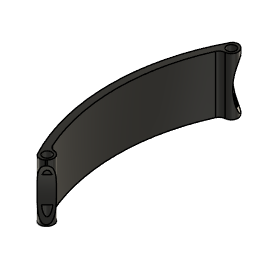
side_coverv6 (Autodesk Fusion 360 design; units mm, degrees)
Autodesk Fusion 360 part; units mm, degrees
note: some values were not read from the file. Set by a fixed rule: which sketch regions a step uses.
sketch "スケッチ1" plane through (0, 0, 2) normal (0, 0, 1) x (-1, 0, 0)
  arc A0 (6.6797, -60.2824) -> (7.9909, -61.0636) centre (8.2815, -59.0848) ccw
  arc A1 (37.5046, -75.2506) -> (7.9909, -61.0636) centre (0, -115.48) ccw
  arc A2 (37.555, -78.1277) -> (37.5046, -75.2506) centre (36.1408, -76.7135) ccw
  line L0 (37.555, -78.1277) -> (34.7247, -80.958)
  arc A3 (31.9509, -81.0106) -> (34.7247, -80.958) centre (33.3105, -79.5438) ccw
  arc A4 (31.9509, -81.0106) -> (-31.9509, -81.0106) centre (0, -115.48) ccw
  arc A5 (-34.7247, -80.958) -> (-31.9509, -81.0106) centre (-33.3105, -79.5438) ccw
  line L1 (-34.7247, -80.958) -> (-37.555, -78.1277)
  arc A6 (-37.5046, -75.2506) -> (-37.555, -78.1277) centre (-36.1408, -76.7135) ccw
  arc A7 (-7.9909, -61.0636) -> (-37.5046, -75.2506) centre (0, -115.48) ccw
  arc A8 (-7.9909, -61.0636) -> (-6.6797, -60.2824) centre (-8.2815, -59.0848) ccw
  arc A9 (-5.0779, -59.48) -> (-6.6797, -60.2824) centre (-5.0779, -61.48) ccw
  line L2 (-5.0779, -59.48) -> (5.0779, -59.48)
  arc A10 (6.6797, -60.2824) -> (5.0779, -59.48) centre (5.0779, -61.48) ccw
  arc A11 (80.8919, -35.1534) -> (72.8829, -37.1429) centre (78.5398, -42.7998) ccw
  line L3 (72.8829, -37.1429) -> (66.8393, -43.1865)
  arc A12 (62.5966, -43.1865) -> (66.8393, -43.1865) centre (64.7179, -41.0652) ccw
  line L4 (62.5966, -43.1865) -> (58.9846, -39.5745)
  arc A13 (58.6276, -32.9007) -> (58.9846, -39.5745) centre (62.5201, -36.039) ccw
  arc A14 (58.6276, -32.9007) -> (58.4491, -29.5638) centre (56.6814, -31.3316) ccw
  line L5 (58.4491, -29.5638) -> (55.679, -26.7937)
  arc A15 (55.2656, -24.5671) -> (55.679, -26.7937) centre (57.0932, -25.3795) ccw
  arc A16 (55.2656, -24.5671) -> (59.7003, -9.6799) centre (0, 0) ccw
  arc A17 (61.6746, -8) -> (59.7003, -9.6799) centre (61.6746, -10) ccw
  line L6 (61.6746, -8) -> (87.43, -8)
  arc A18 (89.417, -10.2273) -> (87.43, -8) centre (87.43, -10) ccw
  arc A19 (83.3318, -33.9973) -> (89.417, -10.2273) centre (0, 0) ccw
  arc A20 (80.8919, -35.1534) -> (83.3318, -33.9973) centre (81.48, -33.2418) ccw
  arc A21 (-80.8919, 35.1534) -> (-72.8829, 37.1429) centre (-78.5398, 42.7998) ccw
  line L7 (-72.8829, 37.1429) -> (-66.8393, 43.1865)
  arc A22 (-62.5966, 43.1865) -> (-66.8393, 43.1865) centre (-64.7179, 41.0652) ccw
  line L8 (-62.5966, 43.1865) -> (-58.9846, 39.5745)
  arc A23 (-58.6276, 32.9007) -> (-58.9846, 39.5745) centre (-62.5201, 36.039) ccw
  arc A24 (-58.6276, 32.9007) -> (-58.4491, 29.5638) centre (-56.6814, 31.3316) ccw
  line L9 (-58.4491, 29.5638) -> (-55.679, 26.7937)
  arc A25 (-55.2656, 24.5671) -> (-55.679, 26.7937) centre (-57.0932, 25.3795) ccw
  arc A26 (-55.2656, 24.5671) -> (-59.7003, 9.6799) centre (0, 0) ccw
  arc A27 (-61.6746, 8) -> (-59.7003, 9.6799) centre (-61.6746, 10) ccw
  line L10 (-61.6746, 8) -> (-87.43, 8)
  arc A28 (-89.417, 10.2273) -> (-87.43, 8) centre (-87.43, 10) ccw
  arc A29 (-83.3318, 33.9973) -> (-89.417, 10.2273) centre (0, 0) ccw
  arc A30 (-80.8919, 35.1534) -> (-83.3318, 33.9973) centre (-81.48, 33.2418) ccw
  arc A31 (-87.43, -5) -> (-92.3976, -10.5682) centre (-87.43, -10) ccw
  arc A32 (-92.3976, -10.5682) -> (-87.3364, -31.9587) centre (0, 0) ccw
  arc A33 (-87.8003, -34.0602) -> (-87.3364, -31.9587) centre (-89.2146, -32.646) ccw
  line L11 (-87.8003, -34.0602) -> (-92.4483, -38.7081)
  arc A34 (-95.7211, -38.0324) -> (-92.4483, -38.7081) centre (-93.8625, -37.2939) ccw
  arc A35 (-95.7211, 38.0324) -> (-95.7211, -38.0324) centre (0, 0) ccw
  arc A36 (-92.4483, 38.7081) -> (-95.7211, 38.0324) centre (-93.8625, 37.2939) ccw
  line L12 (-92.4483, 38.7081) -> (-87.8003, 34.0602)
  arc A37 (-87.3364, 31.9587) -> (-87.8003, 34.0602) centre (-89.2146, 32.646) ccw
  arc A38 (-87.3364, 31.9587) -> (-92.3976, 10.5682) centre (0, 0) ccw
  arc A39 (-92.3976, 10.5682) -> (-87.43, 5) centre (-87.43, 10) ccw
  line L13 (-87.43, 5) -> (-62.273, 5)
  arc A40 (-60.273, 3) -> (-62.273, 5) centre (-62.273, 3) ccw
  line L14 (-60.273, 3) -> (-60.273, -3)
  arc A41 (-62.273, -5) -> (-60.273, -3) centre (-62.273, -3) ccw
  line L15 (-62.273, -5) -> (-87.43, -5)
  arc A42 (-43.4817, -98.8602) -> (-41.4947, -98.0676) centre (-42.8778, -97.4871) ccw
  arc A43 (41.4947, -98.0676) -> (-41.4947, -98.0676) centre (0, -115.48) ccw
  arc A44 (41.4947, -98.0676) -> (43.4817, -98.8602) centre (42.8778, -97.4871) ccw
  arc A45 (43.4817, -98.8602) -> (50.4167, -95.51) centre (0, 0) ccw
  arc A46 (50.4167, -95.51) -> (51.1376, -90.7356) centre (49.0163, -92.8569) ccw
  line L16 (51.1376, -90.7356) -> (40.8708, -80.4688)
  arc A47 (40.8708, -76.2261) -> (40.8708, -80.4688) centre (42.9921, -78.3474) ccw
  line L17 (40.8708, -76.2261) -> (76.2261, -40.8708)
  arc A48 (80.4688, -40.8708) -> (76.2261, -40.8708) centre (78.3474, -42.9921) ccw
  line L18 (80.4688, -40.8708) -> (90.7356, -51.1376)
  arc A49 (90.7356, -51.1376) -> (95.51, -50.4167) centre (92.8569, -49.0163) ccw
  arc A50 (95.51, -50.4167) -> (95.51, 50.4167) centre (0, 0) ccw
  arc A51 (95.51, 50.4167) -> (90.7356, 51.1376) centre (92.8569, 49.0163) ccw
  line L19 (90.7356, 51.1376) -> (80.4688, 40.8708)
  arc A52 (76.2261, 40.8708) -> (80.4688, 40.8708) centre (78.3474, 42.9921) ccw
  line L20 (76.2261, 40.8708) -> (40.8708, 76.2261)
  arc A53 (40.8708, 80.4688) -> (40.8708, 76.2261) centre (42.9921, 78.3474) ccw
  line L21 (40.8708, 80.4688) -> (51.1376, 90.7356)
  arc A54 (51.1376, 90.7356) -> (50.4167, 95.51) centre (49.0163, 92.8569) ccw
  arc A55 (50.4167, 95.51) -> (-50.4167, 95.51) centre (0, 0) ccw
  arc A56 (-50.4167, 95.51) -> (-51.1376, 90.7356) centre (-49.0163, 92.8569) ccw
  line L22 (-51.1376, 90.7356) -> (-40.8708, 80.4688)
  arc A57 (-40.8708, 76.2261) -> (-40.8708, 80.4688) centre (-42.9921, 78.3474) ccw
  line L23 (-40.8708, 76.2261) -> (-76.2261, 40.8708)
  arc A58 (-80.4688, 40.8708) -> (-76.2261, 40.8708) centre (-78.3474, 42.9921) ccw
  line L24 (-80.4688, 40.8708) -> (-90.7356, 51.1376)
  arc A59 (-90.7356, 51.1376) -> (-95.51, 50.4167) centre (-92.8569, 49.0163) ccw
  arc A60 (-95.51, 50.4167) -> (-95.51, -50.4167) centre (0, 0) ccw
  arc A61 (-95.51, -50.4167) -> (-90.7356, -51.1376) centre (-92.8569, -49.0163) ccw
  line L25 (-90.7356, -51.1376) -> (-80.4688, -40.8708)
  arc A62 (-76.2261, -40.8708) -> (-80.4688, -40.8708) centre (-78.3474, -42.9921) ccw
  line L26 (-76.2261, -40.8708) -> (-40.8708, -76.2261)
  arc A63 (-40.8708, -80.4688) -> (-40.8708, -76.2261) centre (-42.9921, -78.3474) ccw
  line L27 (-40.8708, -80.4688) -> (-51.1376, -90.7356)
  arc A64 (-51.1376, -90.7356) -> (-50.4167, -95.51) centre (-49.0163, -92.8569) ccw
  arc A65 (-50.4167, -95.51) -> (-43.4817, -98.8602) centre (0, 0) ccw
  circle A66 centre (37.9314, -81.2868) radius 1.45
  circle A67 centre (-37.9314, -81.2868) radius 1.45
  circle A68 centre (-31.3316, -56.6814) radius 1.65
  circle A69 centre (56.6814, -31.3316) radius 1.65
  circle A70 centre (-39.4713, 89.6381) radius 1.45
  circle A71 centre (89.6381, -39.4713) radius 1.45
  circle A72 centre (-89.6381, -39.4713) radius 1.45
  circle A73 centre (-56.6814, -31.3316) radius 1.65
  circle A74 centre (-31.3316, 56.6814) radius 1.65
  circle A75 centre (31.3316, -56.6814) radius 1.65
  circle A76 centre (56.6814, 31.3316) radius 1.65
  circle A77 centre (39.4713, 89.6381) radius 1.45
  circle A78 centre (89.6381, 39.4713) radius 1.45
  circle A79 centre (-89.6381, 39.4713) radius 1.45
  circle A80 centre (-56.6814, 31.3316) radius 1.65
  circle A81 centre (31.3316, 56.6814) radius 1.65
  circle A82 centre (-48.1818, -92.7295) radius 1.65
  circle A83 centre (55.172, 39.2975) radius 1.65
  circle A84 centre (-42.7658, 42.7658) radius 1.45
  circle A85 centre (42.7658, 42.7658) radius 1.45
  circle A86 centre (-55.172, 39.2975) radius 1.65
  circle A87 centre (48.1818, 92.7295) radius 1.65
  line L28 (-43.1865, -62.5966) -> (-39.5745, -58.9846)
  arc A88 (-32.9007, -58.6276) -> (-39.5745, -58.9846) centre (-36.039, -62.5201) ccw
  arc A89 (-32.9007, -58.6276) -> (-29.5638, -58.4491) centre (-31.3316, -56.6814) ccw
  line L29 (-29.5638, -58.4491) -> (-26.7937, -55.679)
  arc A90 (-24.5671, -55.2656) -> (-26.7937, -55.679) centre (-25.3795, -57.0932) ccw
  arc A91 (-24.5671, -55.2656) -> (-18.2413, -57.6635) centre (0, 0) ccw
  arc A92 (-18.2058, -61.4656) -> (-18.2413, -57.6635) centre (-18.8446, -59.5704) ccw
  arc A93 (-18.2058, -61.4656) -> (-35.435, -70.833) centre (0, -115.48) ccw
  arc A94 (-39.4214, -70.6044) -> (-35.435, -70.833) centre (-37.3, -68.4831) ccw
  line L30 (-39.4214, -70.6044) -> (-43.1865, -66.8393)
  arc A95 (-43.1865, -62.5966) -> (-43.1865, -66.8393) centre (-41.0652, -64.7179) ccw
  line L31 (50.8737, -38.5347) -> (59.0611, -46.7221)
  arc A96 (59.0611, -50.9647) -> (59.0611, -46.7221) centre (56.9398, -48.8434) ccw
  line L32 (59.0611, -50.9647) -> (50.9647, -59.0611)
  arc A97 (46.7221, -59.0611) -> (50.9647, -59.0611) centre (48.8434, -56.9398) ccw
  line L33 (46.7221, -59.0611) -> (38.5347, -50.8737)
  arc A98 (38.7347, -46.4484) -> (38.5347, -50.8737) centre (40.656, -48.7524) ccw
  arc A99 (38.7347, -46.4484) -> (39.0322, -46.1987) centre (0, 0) ccw
  arc A100 (41.8671, -45.628) -> (39.0322, -46.1987) centre (40.9684, -48.4903) ccw
  arc A101 (41.8671, -45.628) -> (45.628, -41.8671) centre (42.7658, -42.7658) ccw
  arc A102 (46.1987, -39.0322) -> (45.628, -41.8671) centre (48.4903, -40.9684) ccw
  arc A103 (46.1987, -39.0322) -> (46.4484, -38.7347) centre (0, 0) ccw
  arc A104 (50.8737, -38.5347) -> (46.4484, -38.7347) centre (48.7524, -40.656) ccw
  circle A105 centre (39.2975, 55.172) radius 1.65
  circle A106 centre (92.7295, -48.1818) radius 1.65
  line L34 (59.0611, 46.7221) -> (50.8737, 38.5347)
  arc A107 (46.4484, 38.7347) -> (50.8737, 38.5347) centre (48.7524, 40.656) ccw
  arc A108 (46.4484, 38.7347) -> (46.1987, 39.0322) centre (0, 0) ccw
  arc A109 (45.628, 41.8671) -> (46.1987, 39.0322) centre (48.4903, 40.9684) ccw
  arc A110 (45.628, 41.8671) -> (41.8671, 45.628) centre (42.7658, 42.7658) ccw
  arc A111 (39.0322, 46.1987) -> (41.8671, 45.628) centre (40.9684, 48.4903) ccw
  arc A112 (39.0322, 46.1987) -> (38.7347, 46.4484) centre (0, 0) ccw
  arc A113 (38.5347, 50.8737) -> (38.7347, 46.4484) centre (40.656, 48.7524) ccw
  line L35 (38.5347, 50.8737) -> (46.7221, 59.0611)
  arc A114 (50.9647, 59.0611) -> (46.7221, 59.0611) centre (48.8434, 56.9398) ccw
  line L36 (50.9647, 59.0611) -> (59.0611, 50.9647)
  arc A115 (59.0611, 46.7221) -> (59.0611, 50.9647) centre (56.9398, 48.8434) ccw
  circle A116 centre (-48.1818, 92.7295) radius 1.65
  circle A117 centre (64.0816, 48.207) radius 1.65
  circle A118 centre (48.1818, -92.7295) radius 1.65
  arc A119 (-89.417, -10.2273) -> (-83.3318, -33.9973) centre (0, 0) ccw
  arc A120 (-87.43, -8) -> (-89.417, -10.2273) centre (-87.43, -10) ccw
  line L37 (-87.43, -8) -> (-61.6746, -8)
  arc A121 (-59.7003, -9.6799) -> (-61.6746, -8) centre (-61.6746, -10) ccw
  arc A122 (-59.7003, -9.6799) -> (-55.2656, -24.5671) centre (0, 0) ccw
  arc A123 (-55.679, -26.7937) -> (-55.2656, -24.5671) centre (-57.0932, -25.3795) ccw
  line L38 (-55.679, -26.7937) -> (-58.4491, -29.5638)
  arc A124 (-58.4491, -29.5638) -> (-58.6276, -32.9007) centre (-56.6814, -31.3316) ccw
  arc A125 (-58.9846, -39.5745) -> (-58.6276, -32.9007) centre (-62.5201, -36.039) ccw
  line L39 (-58.9846, -39.5745) -> (-62.5966, -43.1865)
  arc A126 (-66.8393, -43.1865) -> (-62.5966, -43.1865) centre (-64.7179, -41.0652) ccw
  line L40 (-66.8393, -43.1865) -> (-72.8829, -37.1429)
  arc A127 (-72.8829, -37.1429) -> (-80.8919, -35.1534) centre (-78.5398, -42.7998) ccw
  arc A128 (-83.3318, -33.9973) -> (-80.8919, -35.1534) centre (-81.48, -33.2418) ccw
  circle A129 centre (-64.0816, 48.207) radius 1.65
  circle A130 centre (-39.2975, 55.172) radius 1.65
  circle A131 centre (64.0816, -48.207) radius 1.65
  circle A132 centre (48.207, 64.0816) radius 1.65
  arc A133 (89.417, 10.2273) -> (83.3318, 33.9973) centre (0, 0) ccw
  arc A134 (87.43, 8) -> (89.417, 10.2273) centre (87.43, 10) ccw
  line L41 (87.43, 8) -> (61.6746, 8)
  arc A135 (59.7003, 9.6799) -> (61.6746, 8) centre (61.6746, 10) ccw
  arc A136 (59.7003, 9.6799) -> (55.2656, 24.5671) centre (0, 0) ccw
  arc A137 (55.679, 26.7937) -> (55.2656, 24.5671) centre (57.0932, 25.3795) ccw
  line L42 (55.679, 26.7937) -> (58.4491, 29.5638)
  arc A138 (58.4491, 29.5638) -> (58.6276, 32.9007) centre (56.6814, 31.3316) ccw
  arc A139 (58.9846, 39.5745) -> (58.6276, 32.9007) centre (62.5201, 36.039) ccw
  line L43 (58.9846, 39.5745) -> (62.5966, 43.1865)
  arc A140 (66.8393, 43.1865) -> (62.5966, 43.1865) centre (64.7179, 41.0652) ccw
  line L44 (66.8393, 43.1865) -> (72.8829, 37.1429)
  arc A141 (72.8829, 37.1429) -> (80.8919, 35.1534) centre (78.5398, 42.7998) ccw
  arc A142 (83.3318, 33.9973) -> (80.8919, 35.1534) centre (81.48, 33.2418) ccw
  line L45 (-59.0611, -46.7221) -> (-50.8737, -38.5347)
  arc A143 (-46.4484, -38.7347) -> (-50.8737, -38.5347) centre (-48.7524, -40.656) ccw
  arc A144 (-46.4484, -38.7347) -> (-46.1987, -39.0322) centre (0, 0) ccw
  arc A145 (-45.628, -41.8671) -> (-46.1987, -39.0322) centre (-48.4903, -40.9684) ccw
  arc A146 (-45.628, -41.8671) -> (-41.8671, -45.628) centre (-42.7658, -42.7658) ccw
  arc A147 (-39.0322, -46.1987) -> (-41.8671, -45.628) centre (-40.9684, -48.4903) ccw
  arc A148 (-39.0322, -46.1987) -> (-38.7347, -46.4484) centre (0, 0) ccw
  arc A149 (-38.5347, -50.8737) -> (-38.7347, -46.4484) centre (-40.656, -48.7524) ccw
  line L46 (-38.5347, -50.8737) -> (-46.7221, -59.0611)
  arc A150 (-50.9647, -59.0611) -> (-46.7221, -59.0611) centre (-48.8434, -56.9398) ccw
  line L47 (-50.9647, -59.0611) -> (-59.0611, -50.9647)
  arc A151 (-59.0611, -46.7221) -> (-59.0611, -50.9647) centre (-56.9398, -48.8434) ccw
  circle A152 centre (-55.172, -39.2975) radius 1.65
  circle A153 centre (-39.2975, -55.172) radius 1.65
  circle A154 centre (-42.7658, -42.7658) radius 1.45
  circle A155 centre (92.7295, 48.1818) radius 1.65
  circle A156 centre (48.207, -64.0816) radius 1.65
  circle A157 centre (-64.0816, -48.207) radius 1.65
  circle A158 centre (39.2975, -55.172) radius 1.65
  line L48 (-50.8737, 38.5347) -> (-59.0611, 46.7221)
  arc A159 (-59.0611, 50.9647) -> (-59.0611, 46.7221) centre (-56.9398, 48.8434) ccw
  line L49 (-59.0611, 50.9647) -> (-50.9647, 59.0611)
  arc A160 (-46.7221, 59.0611) -> (-50.9647, 59.0611) centre (-48.8434, 56.9398) ccw
  line L50 (-46.7221, 59.0611) -> (-38.5347, 50.8737)
  arc A161 (-38.7347, 46.4484) -> (-38.5347, 50.8737) centre (-40.656, 48.7524) ccw
  arc A162 (-38.7347, 46.4484) -> (-39.0322, 46.1987) centre (0, 0) ccw
  arc A163 (-41.8671, 45.628) -> (-39.0322, 46.1987) centre (-40.9684, 48.4903) ccw
  arc A164 (-41.8671, 45.628) -> (-45.628, 41.8671) centre (-42.7658, 42.7658) ccw
  arc A165 (-46.1987, 39.0322) -> (-45.628, 41.8671) centre (-48.4903, 40.9684) ccw
  arc A166 (-46.1987, 39.0322) -> (-46.4484, 38.7347) centre (0, 0) ccw
  arc A167 (-50.8737, 38.5347) -> (-46.4484, 38.7347) centre (-48.7524, 40.656) ccw
  circle A168 centre (-48.207, -64.0816) radius 1.65
  arc A169 (-10.2273, 89.417) -> (-33.9973, 83.3318) centre (0, 0) ccw
  arc A170 (-8, 87.43) -> (-10.2273, 89.417) centre (-10, 87.43) ccw
  line L51 (-8, 87.43) -> (-8, 61.6746)
  arc A171 (-9.6799, 59.7003) -> (-8, 61.6746) centre (-10, 61.6746) ccw
  arc A172 (-9.6799, 59.7003) -> (-24.5671, 55.2656) centre (0, 0) ccw
  arc A173 (-26.7937, 55.679) -> (-24.5671, 55.2656) centre (-25.3795, 57.0932) ccw
  line L52 (-26.7937, 55.679) -> (-29.5638, 58.4491)
  arc A174 (-29.5638, 58.4491) -> (-32.9007, 58.6276) centre (-31.3316, 56.6814) ccw
  arc A175 (-39.5745, 58.9846) -> (-32.9007, 58.6276) centre (-36.039, 62.5201) ccw
  line L53 (-39.5745, 58.9846) -> (-43.1865, 62.5966)
  arc A176 (-43.1865, 66.8393) -> (-43.1865, 62.5966) centre (-41.0652, 64.7179) ccw
  line L54 (-43.1865, 66.8393) -> (-37.1429, 72.8829)
  arc A177 (-37.1429, 72.8829) -> (-35.1534, 80.8919) centre (-42.7998, 78.5398) ccw
  arc A178 (-33.9973, 83.3318) -> (-35.1534, 80.8919) centre (-33.2418, 81.48) ccw
  circle A179 centre (-48.207, 64.0816) radius 1.65
  circle A180 centre (55.172, -39.2975) radius 1.65
  circle A181 centre (0, 0) radius 57.48
  circle A182 centre (42.7658, -42.7658) radius 1.45
  circle A183 centre (-92.7295, -48.1818) radius 1.65
  circle A184 centre (-92.7295, 48.1818) radius 1.65
  line L55 (39.5745, -58.9846) -> (43.1865, -62.5966)
  arc A185 (43.1865, -66.8393) -> (43.1865, -62.5966) centre (41.0652, -64.7179) ccw
  line L56 (43.1865, -66.8393) -> (39.4214, -70.6044)
  arc A186 (35.435, -70.833) -> (39.4214, -70.6044) centre (37.3, -68.4831) ccw
  arc A187 (35.435, -70.833) -> (18.2058, -61.4656) centre (0, -115.48) ccw
  arc A188 (18.2413, -57.6635) -> (18.2058, -61.4656) centre (18.8446, -59.5704) ccw
  arc A189 (18.2413, -57.6635) -> (24.5671, -55.2656) centre (0, 0) ccw
  arc A190 (26.7937, -55.679) -> (24.5671, -55.2656) centre (25.3795, -57.0932) ccw
  line L57 (26.7937, -55.679) -> (29.5638, -58.4491)
  arc A191 (29.5638, -58.4491) -> (32.9007, -58.6276) centre (31.3316, -56.6814) ccw
  arc A192 (39.5745, -58.9846) -> (32.9007, -58.6276) centre (36.039, -62.5201) ccw
  arc A193 (10.5682, 92.3976) -> (5, 87.43) centre (10, 87.43) ccw
  line L58 (5, 87.43) -> (5, 62.273)
  arc A194 (3, 60.273) -> (5, 62.273) centre (3, 62.273) ccw
  line L59 (3, 60.273) -> (-3, 60.273)
  arc A195 (-5, 62.273) -> (-3, 60.273) centre (-3, 62.273) ccw
  line L60 (-5, 62.273) -> (-5, 87.43)
  arc A196 (-5, 87.43) -> (-10.5682, 92.3976) centre (-10, 87.43) ccw
  arc A197 (-10.5682, 92.3976) -> (-31.9587, 87.3364) centre (0, 0) ccw
  arc A198 (-34.0602, 87.8003) -> (-31.9587, 87.3364) centre (-32.646, 89.2146) ccw
  line L61 (-34.0602, 87.8003) -> (-38.7081, 92.4483)
  arc A199 (-38.0324, 95.7211) -> (-38.7081, 92.4483) centre (-37.2939, 93.8625) ccw
  arc A200 (38.0324, 95.7211) -> (-38.0324, 95.7211) centre (0, 0) ccw
  arc A201 (38.7081, 92.4483) -> (38.0324, 95.7211) centre (37.2939, 93.8625) ccw
  line L62 (38.7081, 92.4483) -> (34.0602, 87.8003)
  arc A202 (31.9587, 87.3364) -> (34.0602, 87.8003) centre (32.646, 89.2146) ccw
  arc A203 (31.9587, 87.3364) -> (10.5682, 92.3976) centre (0, 0) ccw
  arc A204 (92.3976, -10.5682) -> (87.43, -5) centre (87.43, -10) ccw
  line L63 (87.43, -5) -> (62.273, -5)
  arc A205 (60.273, -3) -> (62.273, -5) centre (62.273, -3) ccw
  line L64 (60.273, -3) -> (60.273, 3)
  arc A206 (62.273, 5) -> (60.273, 3) centre (62.273, 3) ccw
  line L65 (62.273, 5) -> (87.43, 5)
  arc A207 (87.43, 5) -> (92.3976, 10.5682) centre (87.43, 10) ccw
  arc A208 (92.3976, 10.5682) -> (87.3364, 31.9587) centre (0, 0) ccw
  arc A209 (87.8003, 34.0602) -> (87.3364, 31.9587) centre (89.2146, 32.646) ccw
  line L66 (87.8003, 34.0602) -> (92.4483, 38.7081)
  arc A210 (95.7211, 38.0324) -> (92.4483, 38.7081) centre (93.8625, 37.2939) ccw
  arc A211 (95.7211, -38.0324) -> (95.7211, 38.0324) centre (0, 0) ccw
  arc A212 (92.4483, -38.7081) -> (95.7211, -38.0324) centre (93.8625, -37.2939) ccw
  line L67 (92.4483, -38.7081) -> (87.8003, -34.0602)
  arc A213 (87.3364, -31.9587) -> (87.8003, -34.0602) centre (89.2146, -32.646) ccw
  arc A214 (87.3364, -31.9587) -> (92.3976, -10.5682) centre (0, 0) ccw
  arc A215 (35.1534, 80.8919) -> (37.1429, 72.8829) centre (42.7998, 78.5398) ccw
  line L68 (37.1429, 72.8829) -> (43.1865, 66.8393)
  arc A216 (43.1865, 62.5966) -> (43.1865, 66.8393) centre (41.0652, 64.7179) ccw
  line L69 (43.1865, 62.5966) -> (39.5745, 58.9846)
  arc A217 (32.9007, 58.6276) -> (39.5745, 58.9846) centre (36.039, 62.5201) ccw
  arc A218 (32.9007, 58.6276) -> (29.5638, 58.4491) centre (31.3316, 56.6814) ccw
  line L70 (29.5638, 58.4491) -> (26.7937, 55.679)
  arc A219 (24.5671, 55.2656) -> (26.7937, 55.679) centre (25.3795, 57.0932) ccw
  arc A220 (24.5671, 55.2656) -> (9.6799, 59.7003) centre (0, 0) ccw
  arc A221 (8, 61.6746) -> (9.6799, 59.7003) centre (10, 61.6746) ccw
  line L71 (8, 61.6746) -> (8, 87.43)
  arc A222 (10.2273, 89.417) -> (8, 87.43) centre (10, 87.43) ccw
  arc A223 (33.9973, 83.3318) -> (10.2273, 89.417) centre (0, 0) ccw
  arc A224 (35.1534, 80.8919) -> (33.9973, 83.3318) centre (33.2418, 81.48) ccw
  circle A225 centre (0, 0) radius 108
  circle A226 centre (92.7295, -48.1818) radius 3.5
  circle A227 centre (92.7295, 48.1818) radius 3.5
  circle A228 centre (0, 0) radius 104.5
  circle A229 centre (92.7295, -48.1818) radius 2.35
  circle A230 centre (92.7295, 48.1818) radius 2.35
  dimension "d1" = 7
  dimension "d2" = 7
  dimension "d3" = 4.7
  dimension "d4" = 4.7
  constraint coincident A16.centre A19.centre
  constraint concentric A106 A226
  constraint concentric A155 A227
  constraint concentric A16 A228
  constraint coincident A106.centre A228
  constraint concentric A106 A229
  constraint concentric A227 A230
  measures "d1" diameter of A226
  measures "d2" diameter of A227
  measures "d3" diameter of A229
  measures "d4" diameter of A230
extrude "押し出し1" add sketch "スケッチ1" along normal blind 30 contours A49 A50 A225 A226 A228 | L18 A49 A226 A228 | A50 A225 A226 A227 A228 | A226 A228 A229 | A226 A228 A229 | A50 A51 A225 A227 A228 | A227 A228 A230 | A51 L19 A227 A228 | A227 A228 A230 makes body 1
fillet "フィレット1" radius 3.5 2 edges at (-94.291, 45.0494, 17) (-94.291, -45.0494, 17) on bodies 1
sketch "スケッチ2" plane through (0, 0, 32) normal (0, 0, 1) x (-1, 0, 0)
  circle A0 centre (92.7295, 48.1818) radius 2.35
  circle A1 centre (92.7295, -48.1818) radius 2.35
  line L0 (90.2547, -50.6567) -> (90.7356, -51.1376)
  arc A2 (90.7356, -51.1376) -> (95.51, -50.4167) centre (92.8569, -49.0163) ccw
  arc A3 (95.51, -50.4167) -> (95.51, 50.4167) centre (0, 0) ccw
  arc A4 (95.51, 50.4167) -> (90.7356, 51.1376) centre (92.8569, 49.0163) ccw
  line L1 (90.7356, 51.1376) -> (90.2547, 50.6567)
  arc A5 (90.2547, 50.6567) -> (92.472, 44.6913) centre (92.7295, 48.1818) ccw
  arc A6 (95.41, 42.6285) -> (92.472, 44.6913) centre (92.2144, 41.2008) ccw
  arc A7 (95.41, -42.6285) -> (95.41, 42.6285) centre (0, 0) ccw
  arc A8 (92.472, -44.6913) -> (95.41, -42.6285) centre (92.2144, -41.2008) ccw
  arc A9 (92.472, -44.6913) -> (90.2547, -50.6567) centre (92.7295, -48.1818) ccw
  circle A10 centre (92.7295, -48.1818) radius 2.35
  circle A11 centre (92.7295, 48.1818) radius 2.35
  constraint concentric A1 A10
  constraint concentric A0 A11
extrude "押し出し2" add sketch "スケッチ2" along normal blind -8 and the other way blind 22 contours A0 A11 | A1 A10 bodies 1
sketch "スケッチ3" plane through (0, 0, 0) normal (0, 0, 1) x (1, 0, 0)
  circle A0 centre (0, 0) radius 108
  line L0 (0, 0) -> (-76.3675, 76.3675)
  line L1 (0, 0) -> (-108, 0) construction
  line L2 (0, 0) -> (-76.3675, -76.3675)
  line L3 (0, 42.4264) -> (-21.2132, 21.2132)
  line L4 (-21.2132, 21.2132) -> (-42.4264, 0)
  line L5 (-42.4264, 0) -> (0, -42.4264)
  line L6 (0, -42.4264) -> (42.4264, 0)
  line L7 (42.4264, 0) -> (0, 42.4264)
  dimension "d13" = 216
  dimension "d14" = 45
  dimension "d16" = 30
  dimension "d17" = 60
  dimension "d18" = 60
  constraint coincident A0.centre L0.start
  constraint horizontal L1
  constraint coincident A0 L0.end
  constraint coincident A0 L2.end
  constraint perpendicular L0 L2
  constraint coincident L0 L3.end
  constraint perpendicular L0 L3
  constraint perpendicular L0 L4
  constraint perpendicular L4 L5
  constraint perpendicular L5 L6
  constraint perpendicular L3 L7
  measures "d13" diameter of A0
  measures "d14" angle of L0 L1
  measures "d16" distance of L3.end L4.end
  measures "d17" distance of L4.end L5.end
  measures "d18" distance of L5.end L6.end
extrude "押し出し3" add sketch "スケッチ3" along normal blind 32 separate body contours L0 L2 L3 L5 L6 L7 | L0 L2 L4 L5 makes body 2
extrude "押し出し4" cut 1 faces at (0, 0, 0) along direction (0, 0, 1) blind 2 on bodies 2 bodies 2
sketch "スケッチ6" plane through (-21.2132, -21.2132, 0) normal (-0.707107, -0.707107, 0) x (0.707107, -0.707107, 0)
  line L0 (-30, 2) -> (30, 2)
  line L1 (30, 2) -> (30, 32)
  line L2 (30, 32) -> (-30, 32)
  line L3 (-30, 32) -> (-30, 2)
  line L4 (30, 32) -> (-30, 2)
  line L5 (30, 2) -> (-30, 32)
  line L6 (0, 17) -> (0, 16)
  circle A0 centre (0, 16) radius 31
  dimension "d29" = 1
  dimension "d30" = 62
  constraint coincident L1.end L2.start
  constraint coincident L0.start L3.end
  constraint coincident L0.end L1.start
  constraint coincident L2.end L3.start
  constraint vertical L6
  constraint coincident L6.end A0.centre
  measures "d29" distance of L6.start L6.end
  measures "d30" diameter of A0
extrude "押し出し5" cut sketch "スケッチ6" along normal blind 95 contours L0 L4 L5 A0 | L0 A0 | L3 A0 | L3 L4 L5 A0 | L0 L5 A0 | L2 L4 L5 A0 | L1 L4 L5 A0 | L1 L5 A0 | L2 L4 A0 | L1 L4 A0 | L1 A0 | L2 A0 bodies 1
sketch "スケッチ8" plane through (-21.2132, 21.2132, 0) normal (-0.707107, 0.707107, 0) x (-0.707107, -0.707107, 0)
  line L0 (-30, 2) -> (30, 2)
  line L1 (30, 2) -> (30, 32)
  line L2 (30, 32) -> (-30, 32)
  line L3 (-30, 32) -> (-30, 2)
  line L4 (-30, 32) -> (30, 2)
  line L5 (30, 32) -> (-30, 2)
  line L6 (0, 17) -> (0, 16)
  circle A0 centre (0, 16) radius 31
  dimension "d31" = 1
  dimension "d32" = 62
  constraint coincident L2.end L3.start
  constraint coincident L0.end L1.start
  constraint coincident L1.end L2.start
  constraint coincident L0.start L3.end
  constraint vertical L6
  constraint coincident L6.end A0.centre
  measures "d31" distance of L6.start L6.end
  measures "d32" diameter of A0
extrude "押し出し6" cut sketch "スケッチ8" along normal blind 120 contours L0 L4 L5 A0 | L0 A0 | L1 L4 L5 A0 | L2 L4 L5 A0 | L1 A0 | L2 A0 bodies 1
hidden bodies 2
